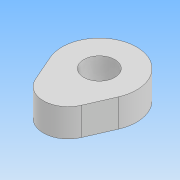
# Autodesk Inventor part: 偏心倫
Saved by Autodesk Inventor 2021 (Build 250183000, 183)
## iProperties
Created: 2025-12-12
Part Number: 偏心倫
Material: 一般
Document SubType Name: Modeling
Designer: User
Density: 1 g/cm^3
Appearance: 預設
Author: User
Autodesk Inventor part; units mm, degrees
ref_plane "YZ Plane" through (0, 0, 0) normal (1, 0, 0) x (0, 1, 0)
ref_plane "XZ Plane" through (0, 0, 0) normal (0, 1, 0) x (-1, 0, 0)
ref_plane "XY Plane" through (0, 0, 0) normal (0, 0, 1) x (1, 0, 0)
sketch "草圖1" plane through (0, 0, 0) normal (0, 1, 0) x (-1, 0, 0)
  circle A0 centre (0, 0) radius 25
  circle A1 centre (0, 50) radius 40
  line L0 (0, 90) -> (52.1614, 90)
  circle A2 centre (0, 0) radius 60
  line L1 (0, -60) -> (92.0478, -60)
  line L2 (36.6606, 66) -> (54.9909, 24)
  line L3 (-54.9909, 24) -> (-36.6606, 66)
  dimension "d0" = 50
  dimension "d4" = 120
  dimension "d5" = 80
  dimension "d7" = 50
  constraints: 8 end point, 6 point on circle, 6 tangent, 3 centre point, 2 horizontal, 1 coincident, 1 vertical alignment
  measures "d0" diameter of A0
  measures "d4" diameter of A2
  measures "d5" diameter of A1
  measures "d7" distance of A0.centre A1.centre
extrude "擠出1" add sketch "草圖1" along normal blind 45 contours A0 A1 A2 | A0 A1 A2 | A2 A1 | A1 L2 A2 | A2 L3 A1
